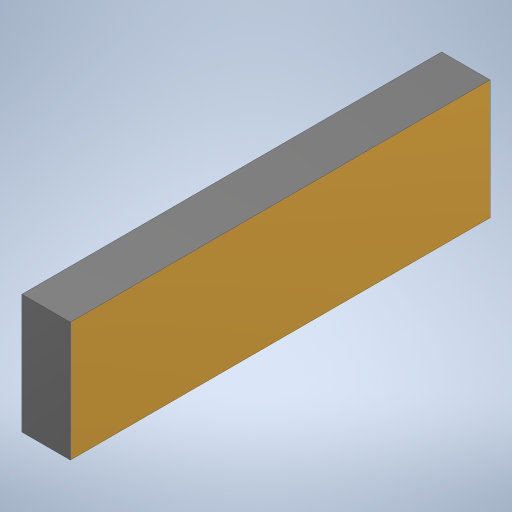
# Autodesk Inventor part: cupboard
Saved by Autodesk Inventor 2023 (Build 270158000, 158)
## iProperties
Created: 2022-09-12
Part Number: cupboard
Material: 常规
Document SubType Name: Modeling
Designer: byfbi
Density: 1 g/cm^3
Appearance: 默认
Author: byfbi
Autodesk Inventor part; units mm, degrees
ref_plane "YZ Plane" through (0, 0, 0) normal (1, 0, 0) x (0, 1, 0)
ref_plane "XZ Plane" through (0, 0, 0) normal (0, 1, 0) x (-1, 0, 0)
ref_plane "XY Plane" through (0, 0, 0) normal (0, 0, 1) x (1, 0, 0)
sketch "草图1" plane through (0, 0, 0) normal (1, 0, 0) x (0, 1, 0)
  line L0 (370, -1300) -> (-370, -1300)
  line L1 (-370, -1300) -> (-370, 1300)
  line L2 (-370, 1300) -> (370, 1300)
  line L3 (370, 1300) -> (370, -1300)
  line L4 (370, -1300) -> (-370, 1300) construction
  line L5 (-370, -1300) -> (370, 1300) construction
  point P0 (0, 0)
  dimension "d0" = 740
  dimension "d1" = 2600
  constraints: 12 end point, 2 midpoint, 2 parallel, 1 horizontal, 1 perpendicular
  measures "d0" distance of L1.end L2.end
  measures "d1" distance of L0.end L1.end
extrude "拉伸1" add sketch "草图1" along normal blind 300
